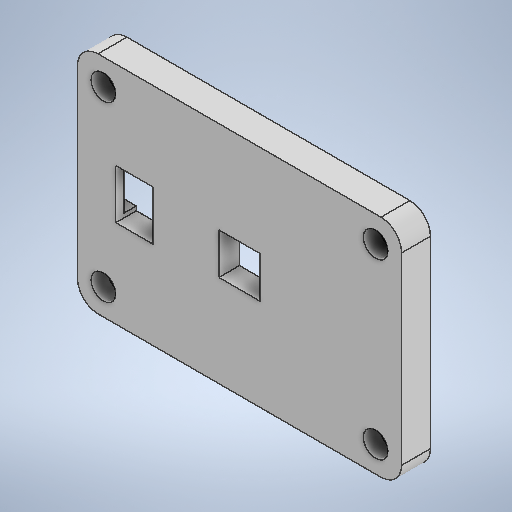
# Autodesk Inventor part: lid
Saved by Autodesk Inventor 2025 (Build 290162000, 162)
## iProperties
Created: 2026-02-25
Part Number: lid
Material: 一般
Document SubType Name: Modeling
Designer: sooo1
Density: 1 g/cm^3
Appearance: 既定
Author: sooo1
Autodesk Inventor part; units mm, degrees
ref_plane "YZ Plane" through (0, 0, 0) normal (1, 0, 0) x (0, 1, 0)
ref_plane "XZ Plane" through (0, 0, 0) normal (0, 1, 0) x (-1, 0, 0)
ref_plane "XY Plane" through (0, 0, 0) normal (0, 0, 1) x (1, 0, 0)
sketch "スケッチ1" plane through (0, 0, 0) normal (0, 0, 1) x (1, 0, 0)
  line L0 (-39.3, -27.3) -> (39.3, -27.3) construction
  line L1 (39.3, 27.3) -> (39.3, -27.3) construction
  line L2 (-39.3, 27.3) -> (39.3, 27.3) construction
  line L3 (-39.3, 27.3) -> (-39.3, 5) construction
  line L4 (36.3, 24.3) -> (36.3, -24.3) construction
  line L5 (36.3, -24.3) -> (-36.3, -24.3) construction
  line L6 (-36.3, -24.3) -> (-36.3, -5) construction
  line L7 (-36.3, 24.3) -> (36.3, 24.3) construction
  line L8 (39.3, 27.3) -> (-39.3, 27.3)
  line L9 (-39.3, 27.3) -> (-39.3, -27.3)
  line L10 (-39.3, -27.3) -> (39.3, -27.3)
  line L11 (39.3, -27.3) -> (39.3, 27.3)
  line L12 (36.3, -24.3) -> (-36.3, -24.3)
  line L13 (-36.3, -24.3) -> (-36.3, 24.3)
  line L14 (-36.3, 24.3) -> (36.3, 24.3)
  line L15 (36.3, 24.3) -> (36.3, -24.3)
  line L16 (4, -4) -> (4, 4) construction
  line L17 (-4, -4) -> (4, -4) construction
  line L18 (-4, 4) -> (-4, -4) construction
  line L19 (4, 4) -> (-4, 4) construction
  line L20 (-22, 5) -> (-29, 5) construction
  line L21 (-29, -5) -> (-22, -5) construction
  line L22 (5, 5) -> (5, -5)
  line L23 (5, -5) -> (-5, -5)
  line L24 (-5, -5) -> (-5, 5)
  line L25 (-5, 5) -> (5, 5)
  line L26 (-2, 2) -> (-2, -2) construction
  line L27 (-2, -2) -> (2, -2) construction
  line L28 (2, -2) -> (2, 2) construction
  line L29 (2, 2) -> (-2, 2) construction
  line L30 (-36.3, -5) -> (-39.3, -5) construction
  line L31 (-39.3, -5) -> (-39.3, -27.3) projected
  line L32 (-39.3, 5) -> (-36.3, 5) construction
  line L33 (-36.3, 5) -> (-36.3, 24.3) projected
  line L34 (-36.3, 5) -> (-39.3, 5)
  line L35 (-36.3, -5) -> (-39.3, -5)
  circle A0 centre (-33, 21) radius 1.6 projected
  circle A1 centre (-33, -21) radius 1.6 projected
  circle A2 centre (33, -21) radius 1.6 projected
  circle A3 centre (33, 21) radius 1.6 projected
  line L36 (-22, -5) -> (-22, 5) construction
  line L37 (-29, 5) -> (-29, -5) construction
  line L38 (-21, 6) -> (-30, 6)
  line L39 (-30, 6) -> (-30, -6)
  line L40 (-30, -6) -> (-21, -6)
  line L41 (-21, -6) -> (-21, 6)
  circle A4 centre (33, -21) radius 3
  circle A5 centre (33, 21) radius 3
  circle A6 centre (-33, 21) radius 3
  circle A7 centre (-33, -21) radius 3
  line L42 (-36.3, 14.3) -> (-26.3, 14.3) projected
  line L43 (-26.3, 14.3) -> (-26.3, 24.3) projected
  line L44 (-36.3, -14.3) -> (-26.3, -14.3) projected
  line L45 (-26.3, -14.3) -> (-26.3, -24.3) projected
  line L46 (26.3, 14.3) -> (26.3, 24.3) projected
  line L47 (36.3, 14.3) -> (26.3, 14.3) projected
  line L48 (26.3, -14.3) -> (26.3, -24.3) projected
  line L49 (36.3, -14.3) -> (26.3, -14.3) projected
  line L50 (-36.3, 5) -> (-30, 5)
  line L51 (-36.3, -5) -> (-30, -5)
  point P0 (0, 0)
  dimension "d4" = 1
  dimension "d7" = 1
  dimension "d10" = 6
  constraints: 40 end point, 6 collinear, 6 point on line, 5 perpendicular, 4 centre point, 4 parallel, 3 equal radius, 3 horizontal, 6 other
  measures "d4" distance between parallel lines of L16 L22
  measures "d7" distance between parallel lines of L36 L41
  measures "d10" diameter of A4
extrude "押し出し1" add sketch "スケッチ1" along normal blind 3 contours L11 L10 L9 L35 L13 L12 L15 L14 L34 L8 | L34 L13 L35 L9 | L50 L39 L51 L13 | L13 L42 L43 L14 L46 L47 L15 L49 L48 L12 L45 L44 L51 L39 L40 L41 L38 L50 | L13 L14 L43 L42 | L44 L45 L12 L13 | L14 L15 L47 L46 | L48 L49 L15 L12 | A4 | A5 | A6 | A7
extrude "押し出し3" add sketch "スケッチ1" along normal blind 4 from surface at 3 contours L11 L10 L9 L35 L13 L12 L15 L14 L34 L8 | L34 L13 L35 L9 | L50 L39 L51 L13 | L13 L42 L43 L14 L46 L47 L15 L49 L48 L12 L45 L44 L51 L39 L40 L41 L38 L50 | L13 L14 L43 L42 | L44 L45 L12 L13 | L14 L15 L47 L46 | L48 L49 L15 L12
extrude "押し出し4" cut sketch "スケッチ1" along normal blind 2 contours L50 L39 L51 L13 | L13 L42 L43 L14 L46 L47 L15 L49 L48 L12 L45 L44 L51 L39 L40 L41 L38 L50
extrude "押し出し2" cut sketch "スケッチ1" along normal blind 5 contours L34 L13 L35 L9 | L50 L39 L51 L13
sketch "スケッチ2" plane through (0, 0, 0) normal (0, 0, -1) x (-1, 0, 0)
  line L0 (36.3, -24.3) -> (36.3, 24.3) projected
  line L1 (36.3, 24.3) -> (-36.3, 24.3) projected
  line L2 (26.3, 24.3) -> (26.3, 14.3) projected
  line L3 (26.3, 14.3) -> (36.3, 14.3) projected
  line L4 (36.3, -14.3) -> (26.3, -14.3) projected
  line L5 (26.3, -14.3) -> (26.3, -24.3) projected
  line L6 (-36.3, -24.3) -> (36.3, -24.3) projected
  line L7 (36.3, -24.3) -> (36.3, -5) construction
  line L8 (-26.3, -14.3) -> (-36.3, -14.3) projected
  line L9 (-26.3, -24.3) -> (-26.3, -14.3) projected
  line L10 (-36.3, 24.3) -> (-36.3, -24.3) projected
  line L11 (-36.3, 14.3) -> (-26.3, 14.3) projected
  line L12 (-26.3, 14.3) -> (-26.3, 24.3) projected
  circle A0 centre (33, 21) radius 1.6 projected
  circle A1 centre (33, -21) radius 1.6 projected
  circle A2 centre (-33, 21) radius 1.6 projected
  circle A3 centre (-33, -21) radius 1.6 projected
  line L13 (36.3, 24) -> (-36.3, 24)
  line L14 (36, -24.3) -> (36, 24.3)
  line L15 (36.3, -24) -> (-36.3, -24)
  line L16 (-36, 24.3) -> (-36, -24.3)
  point P0 (0, 0)
  point P1 (-36, -14.3)
  point P2 (-36, -24)
  point P3 (-26.3, -24)
  point P4 (-36, 24)
  point P5 (-36, 14.3)
  point P6 (-26.3, 24)
  point P7 (26.3, -24)
  point P8 (36, -24)
  point P9 (36, -14.3)
  point P10 (36, 14.3)
  point P11 (36, 24)
  point P12 (26.3, 24)
  dimension "d17" = 0.3
  dimension "d18" = 0.3
  dimension "d19" = 0.3
  dimension "d20" = 0.3
  constraints: 8 end point, 5 point on line, 3 perpendicular, 1 parallel
  measures "d17" distance between parallel lines of L1 L13
  measures "d18" distance between parallel lines of L0 L14
  measures "d19" distance between parallel lines of L6 L15
  measures "d20" distance between parallel lines of L10 L16
extrude "押し出し5" add sketch "スケッチ2" along normal blind 1 contours L15 L5 L4 L14 | L3 L2 L13 L14 | L15 L16 L8 L9 | L12 L11 L16 L13
fillet "フィレット1" radius 5 4 edges at (-39.3, -27.3, 3.5) (-39.3, 27.3, 3.5) (39.3, -27.3, 3.5) (39.3, 27.3, 3.5)
